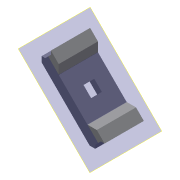
# Autodesk Inventor part: 20_Cube_Insert_Mirror_Holder_wLogo_v3
Saved by Autodesk Inventor 2022 (Build 260153000, 153)
## iProperties
Created: 2019-07-22
Part Number: 20_Cube_Insert_Mirror_Holder_wLogo_v3
Material: Generic
Document SubType Name: Modeling
Designer: diederichbenedict
Density: 1 g/cm^3
Appearance: Default
Mass: 13.6419 g
Surface Area: 50.8514 cm^2
Volume: 13.6419 cm^3
Author: diederichbenedict
Autodesk Inventor part; units mm, degrees
ref_plane "YZ Plane" through (0, 0, 0) normal (1, 0, 0) x (0, 1, 0)
ref_plane "XZ Plane" through (0, 0, 0) normal (0, 1, 0) x (-1, 0, 0)
ref_plane "XY Plane" through (0, 0, 0) normal (0, 0, 1) x (1, 0, 0)
sketch "Sketch1" plane through (0, 0, 0) normal (0, 0, 1) x (1, 0, 0)
  line L0 (-16.8009, 21.2415) -> (21.2415, -16.8009)
  line L1 (21.2415, -16.8009) -> (16.8009, -21.2415)
  line L2 (16.8009, -21.2415) -> (-21.2415, 16.8009)
  line L3 (-21.2415, 16.8009) -> (-16.8009, 21.2415)
  line L4 (-16.8009, 21.2415) -> (16.8009, -21.2415) construction
  line L5 (21.2415, -16.8009) -> (-21.2415, 16.8009) construction
  line L6 (-16.8009, 21.2415) -> (36.9991, 21.2415) construction
  line L7 (-21.2415, 16.8009) -> (-24, 16.8009)
  line L8 (16.8009, -21.2415) -> (16.8009, -24)
  line L9 (16.8009, -24) -> (-24, 16.8009)
  line L10 (-16.8009, 21.2415) -> (-16.8009, 24)
  line L11 (21.2415, -16.8009) -> (24, -16.8009)
  line L12 (24, -16.8009) -> (-16.8009, 24)
  line L13 (-24, 16.8009) -> (-24, 12.6863)
  line L14 (16.8009, -24) -> (12.6863, -24)
  line L15 (-24, 12.6863) -> (12.6863, -24)
  line L16 (-24, 16.8009) -> (-11.8721, 28.9288) construction
  line L17 (-24, 16.8009) -> (-6.8486, 16.8009) construction
  point P0 (0, 0)
  dimension "d0" = 53.8
  dimension "d1" = 45
  dimension "d2" = 6.28
  dimension "d5" = 8
  dimension "d72" = 24
  dimension "d73" = 45
  constraints: 36 end point, 9 parallel, 2 equal length, 2 horizontal, 2 midpoint, 2 perpendicular, 1 point on line, 1 vertical
  measures "d0" distance of L0.start L0.end
  measures "d1" angle of L0 L6
  measures "d2" distance of L0.end L1.end
  measures "d5" distance from line of L15 point (0, 0)
  measures "d72" distance from line of point (0, 0) L13
  measures "d73" angle of L17 L16
extrude "Extrusion1" add sketch "Sketch1" along normal blind 30
ref_plane "Work Plane1" through (16.9, -16.9, -8) normal (-0.7071, -0.7071, 0) x (0, 0, 1)
sketch "Sketch7" plane through (0, 0, 30) normal (0, 0, 1) x (1, 0, 0)
  line L0 (21.2415, -16.8009) -> (24, -16.8009) projected
  line L1 (24, -16.8009) -> (-16.8009, 24) projected
  line L2 (-16.8009, 24) -> (-16.8009, 21.2415) projected
  line L3 (-16.8009, 21.2415) -> (-21.2415, 16.8009) projected
  line L4 (-21.2415, 16.8009) -> (-24, 16.8009) projected
  line L5 (-24, 16.8009) -> (-24, 12.6863) projected
  line L6 (-24, 12.6863) -> (12.6863, -24) projected
  line L7 (12.6863, -24) -> (16.8009, -24) projected
  line L8 (16.8009, -24) -> (16.8009, -21.2415) projected
  line L9 (16.8009, -21.2415) -> (21.2415, -16.8009) projected
  line L10 (3.5996, 3.5996) -> (-5.6569, -5.6569)
  line L11 (-24, 12.6863) -> (12.6863, -24) projected
  line L12 (18.1593, -3.761) -> (10.9602, -10.9602)
  line L13 (10.9602, -10.9602) -> (-10.9602, 10.9602)
  line L14 (-10.9602, 10.9602) -> (-3.761, 18.1593)
  line L15 (-3.761, 18.1593) -> (18.1593, -3.761)
  line L16 (18.1593, -3.761) -> (-10.9602, 10.9602) construction
  line L17 (10.9602, -10.9602) -> (-3.761, 18.1593) construction
  line L18 (-10.9602, 10.9602) -> (-10.9602, 18.1593)
  line L19 (24, -16.8009) -> (-16.8009, 24) projected
  line L20 (10.9602, -10.9602) -> (18.1593, -10.9602)
  point P0 (0, 0)
  dimension "d28" = 31
  dimension "d29" = 0
  dimension "d74" = 0
  constraints: 18 end point, 4 midpoint, 2 parallel, 2 perpendicular, 2 point on line, 1 vertical
  measures "d28" distance of L12.end L13.end
  measures "d29" distance from line of L13 point (0, 0)
  measures "d74" angle of L1 L15
extrude "Extrusion7" cut sketch "Sketch7" against normal through all contours L20 L12 L1 | L12 L13 L10 L1 | L1 L14 L15 L12 | L10 L13 L14 L1 | L14 L18 L1
sketch "Sketch13" plane through (0, 0, 30) normal (0, 0, 1) x (1, 0, 0)
  line L0 (-10.9602, 18.1593) -> (-16.8009, 24) construction
  line L1 (-16.8009, 24) -> (-16.8009, 21.2415) projected
  line L2 (-16.8009, 21.2415) -> (-21.2415, 16.8009) projected
  line L3 (-21.2415, 16.8009) -> (-24, 16.8009) projected
  line L4 (-24, 16.8009) -> (-24, 12.6863) construction
  line L5 (-24, 12.6863) -> (12.6863, -24) construction
  line L6 (12.6863, -24) -> (16.8009, -24) construction
  line L7 (16.8009, -24) -> (16.8009, -21.2415) projected
  line L8 (16.8009, -21.2415) -> (21.2415, -16.8009) projected
  line L9 (21.2415, -16.8009) -> (24, -16.8009) projected
  line L10 (24.1, -24.6971) -> (24.1, -16.7029) construction
  line L11 (24.1, -16.7029) -> (-16.9409, 24.338) construction
  line L12 (-16.9409, 24.338) -> (-16.9409, 21.2995)
  line L13 (-16.9409, 21.2995) -> (-21.2995, 16.9409)
  line L14 (-21.2995, 16.9409) -> (-24.14, 16.9409)
  line L15 (-24.14, 16.9409) -> (-24.14, 12.6283) construction
  line L16 (-24.14, 12.6283) -> (12.6283, -24.14) construction
  line L17 (12.6283, -24.14) -> (16.9409, -24.14) construction
  line L18 (16.9409, -24.14) -> (16.9409, -21.2995)
  line L19 (16.9409, -21.2995) -> (21.2995, -16.9409)
  line L20 (21.2995, -16.9409) -> (24.2814, -16.9409)
  line L21 (24.2814, -16.9409) -> (53.8994, -46.5588) construction
  line L22 (53.8994, -46.5588) -> (45.9617, -46.5588) construction
  line L23 (45.9617, -46.5588) -> (24.1, -24.6971) construction
  line L24 (16.8009, -24) -> (16.9409, -24)
  line L25 (24, -16.8009) -> (24.1393, -16.9409)
  line L26 (-21.2415, 16.8009) -> (-22.9, 16.8009) projected
  line L27 (18.1593, -10.9602) -> (10.9602, -10.9602) projected
  line L28 (10.9602, -10.9602) -> (-10.9602, 10.9602) projected
  line L29 (-10.9602, 10.9602) -> (-10.9602, 18.1593) projected
  line L30 (24, -16.8009) -> (18.1593, -10.9602) projected
  line L31 (-24, 12.6863) -> (-24, 16.8009) projected
  line L32 (-24, 16.8009) -> (-24, 16.9409)
  line L33 (-16.8009, 24) -> (-16.9409, 24.14)
  point P0 (0, 0)
  point P1 (-22.9, 16.9409)
  dimension "d93" = 0.14
  constraints: 36 end point, 6 point on line, 1 collinear, 1 perpendicular, 9 other
  measures "d93" distance between parallel lines of L2 L13
extrude "IM_offset" add sketch "Sketch13" against normal up to surface (30 mm away)
sketch "Skizze14" plane through (12.6863, -24, 30) normal (-0.7071, -0.7071, 0) x (-0.7071, 0.7071, 0)
  line L0 (21.8411, 19.1) -> (30.0411, 19.1)
  line L1 (30.0411, 19.1) -> (30.0411, 10.9)
  line L2 (30.0411, 10.9) -> (21.8411, 10.9)
  line L3 (21.8411, 10.9) -> (21.8411, 19.1)
  line L4 (21.8411, 19.1) -> (30.0411, 10.9) construction
  line L5 (30.0411, 19.1) -> (21.8411, 10.9) construction
  line L6 (0, 30) -> (0, 0) construction
  line L7 (51.8823, 30) -> (51.8823, 0) construction
  line L8 (0, 30) -> (51.8823, 0) construction
  line L9 (51.8823, 0) -> (51.8823, 30) construction
  line L10 (51.8823, 30) -> (0, 0) construction
  line L11 (-2.9094, 0) -> (5.3506, 0) construction
  point P0 (25.9411, 30)
  point P1 (25.9411, 15)
  dimension "d94" = 8.2
  dimension "d95" = 8.2
  constraints: 18 end point, 3 equal length, 3 midpoint, 1 horizontal, 1 perpendicular, 1 point on line
  measures "d94" distance of L1.end L2.end
  measures "d95" distance of L0.end L1.end
extrude "Extrusion11" cut sketch "Skizze14" against normal blind 10
sketch "Skizze15" plane through (12.6863, -24, 30) normal (-0.7071, -0.7071, 0) x (-0.7071, 0.7071, 0)
  line L0 (30.0411, 19.1) -> (30.0411, 10.9) projected
  line L1 (30.0411, 10.9) -> (21.8411, 10.9) projected
  line L2 (21.8411, 10.9) -> (21.8411, 19.1) projected
  line L3 (21.8411, 19.1) -> (30.0411, 19.1) projected
  line L4 (0, 30) -> (51.8823, 30) projected
  line L5 (0, 30) -> (0, 0) projected
  line L6 (51.8823, 0) -> (0, 0) projected
  line L7 (51.8823, 30) -> (51.8823, 0) projected
  line L8 (51.8823, 30) -> (51.8823, 0) projected
  line L9 (0, 30) -> (0, 0) projected
  line L10 (51.8823, 30) -> (0, 0)
  line L11 (0, 0) -> (0, 30)
  line L12 (-2.9094, 30) -> (5.3506, 30) projected
  line L13 (51.8823, 0) -> (0, 30)
  line L14 (38.4411, 2.5) -> (13.4411, 2.5)
  line L15 (13.4411, 2.5) -> (13.4411, 27.5)
  line L16 (13.4411, 27.5) -> (38.4411, 27.5)
  line L17 (38.4411, 27.5) -> (38.4411, 2.5)
  line L18 (38.4411, 2.5) -> (13.4411, 27.5) construction
  line L19 (13.4411, 2.5) -> (38.4411, 27.5) construction
  point P0 (25.9411, 30)
  point P1 (25.9411, 15)
  dimension "d98" = 25
  dimension "d99" = 25
  constraints: 18 end point, 3 midpoint, 2 parallel, 2 perpendicular, 1 horizontal
  measures "d98" distance of L15.end L16.end
  measures "d99" distance of L14.end L15.end
extrude "Extrusion12" cut sketch "Skizze15" against normal blind 3 contours L3 L2 L13 L15 L16 L17 L10 L0 | L10 L17 L13 L0 | L13 L17 L14 L15 L10 L2 L1 L0 | L2 L10 L15 L13
chamfer "Fase1" distance 2.5 angle 45 4 edges at (3.182, -14.4957, 15) (-5.6569, -5.6569, 27.5) (-14.4957, 3.182, 15) (-5.6569, -5.6569, 2.5)
equation "\"d3\" = MirrorThickness1"
equation "\"MirrorThickness1\" = 30"
body "Solid1"
